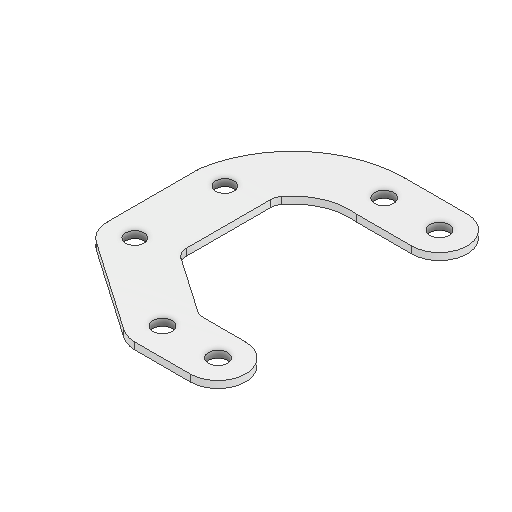
# Autodesk Inventor part: Rear Gusset
Saved by Autodesk Inventor 2025 (Build 290162000, 162)
## iProperties
Created: 2025-02-12
Part Number: Rear Gusset
Material: Acetal Resin, White
Document SubType Name: Modeling
Designer: Averey Ku
Density: 1.425 g/cm^3
Appearance: Smooth - White
Author: Averey Ku
Autodesk Inventor part; units mm, degrees
ref_plane "YZ Plane" through (0, 0, 0) normal (1, 0, 0) x (0, 1, 0)
ref_plane "XZ Plane" through (0, 0, 0) normal (0, 1, 0) x (-1, 0, 0)
ref_plane "XY Plane" through (0, 0, 0) normal (0, 0, 1) x (1, 0, 0)
sketch "gusset" plane through (0, 0, 0) normal (0, 0, 1) x (1, 0, 0)
  circle A0 centre (-8.9225, 14.8571) radius 2.1844
  circle A1 centre (-21.6225, 14.8571) radius 2.1844
  arc A2 (-21.6225, 21.2071) -> (-21.6225, 8.5071) centre (-21.6225, 14.8571) ccw
  arc A3 (-5.308, 20.078) -> (-8.9225, 21.2071) centre (-8.9225, 14.8571) ccw
  line L0 (18.065, 0.5696) -> (18.065, -20.0679)
  line L1 (3.7775, -22.5548) -> (3.7775, -3.322)
  line L2 (2.4097, -0.7116) -> (-10.0906, 7.9425)
  line L3 (-21.6225, 8.5071) -> (-11.8979, 8.5071)
  line L4 (-21.6225, 21.2071) -> (-8.9225, 21.2071)
  arc A4 (18.065, 0.5696) -> (15.3295, 5.7905) centre (11.715, 0.5696) ccw
  line L5 (-5.308, 20.078) -> (15.3295, 5.7905)
  circle A5 centre (-21.6232, -35.9429) radius 2.1844
  circle A6 centre (-8.9225, -35.9429) radius 2.1844
  line L6 (-21.6246, -29.5943) -> (-8.9205, -29.5916)
  line L7 (-21.6233, -42.2916) -> (-7.3358, -42.2916)
  arc A7 (-21.6246, -29.5943) -> (-21.6233, -42.2916) centre (-21.6232, -35.9429) ccw
  circle A8 centre (11.715, 0.5696) radius 2.0955
  circle A9 centre (11.715, -20.0679) radius 2.0955
  arc A10 (3.7775, -3.322) -> (2.4097, -0.7116) centre (0.6025, -3.322) ccw
  arc A11 (-10.0906, 7.9425) -> (-11.8979, 8.5071) centre (-11.8979, 5.3321) ccw
  arc A12 (-7.3358, -42.2916) -> (17.9607, -21.2138) centre (-7.3358, -16.5727) ccw
  arc A13 (17.9607, -21.2138) -> (18.065, -20.0679) centre (11.715, -20.0679) ccw
  arc A14 (-8.9205, -29.5916) -> (3.1382, -24.4655) centre (-7.3358, -16.5727) ccw
  arc A15 (3.1382, -24.4655) -> (3.7775, -22.5548) centre (0.6025, -22.5548) ccw
  point P0 (-7.0147, -10.522)
  point P1 (18.065, -20.6044)
  point P2 (3.7775, -23.5365)
  point P3 (5.0107, 12.9342)
  dimension "d0" = 12.7
  dimension "d2" = 14.2875
  dimension "d3" = 4.191
  dimension "d4" = 3.175
  dimension "d8" = 12.7
  dimension "d12" = 14.2875
  dimension "d13" = 6.35
  dimension "d14" = 15.875
  dimension "d15" = 3.175
  measures "d0" diameter of A4
  measures "d3" diameter of A8
  measures "d4" radius of A10
  measures "d8" distance from line of L2 point (5.011, 12.934)
  measures "d12" distance of L7.start L7.end
  measures "d13" radius of A13
  measures "d14" vertical distance of A6.centre A9.centre
  measures "d15" radius of A15
sketch "Sketch1" plane through (0, 0, 0) normal (0, 1, 0) x (-1, 0, 0)
  circle A0 centre (12.7, 0) radius 2.1844
  circle A1 centre (0, 0) radius 2.1844
  arc A2 (0, 6.35) -> (0, -6.35) centre (0, 0) ccw
  arc A3 (16.3145, 5.2209) -> (12.7, 6.35) centre (12.7, 0) ccw
  line L0 (39.6875, -14.2875) -> (39.6875, -34.925)
  line L1 (25.4, -37.4118) -> (25.4, -18.1791)
  line L2 (24.0322, -15.5687) -> (11.5319, -6.9145)
  line L3 (0, -6.35) -> (9.7246, -6.35)
  line L4 (0, 6.35) -> (12.7, 6.35)
  arc A4 (39.6875, -14.2875) -> (36.952, -9.0666) centre (33.3375, -14.2875) ccw
  line L5 (16.3145, 5.2209) -> (36.952, -9.0666)
  circle A5 centre (-0.0007, -50.8) radius 2.1844
  circle A6 centre (12.7, -50.8) radius 2.1844
  line L6 (-0.0021, -44.4514) -> (12.702, -44.4486)
  line L7 (-0.0008, -57.1486) -> (14.2867, -57.1486)
  arc A7 (-0.0021, -44.4514) -> (-0.0008, -57.1486) centre (-0.0007, -50.8) ccw
  circle A8 centre (33.3375, -14.2875) radius 2.0955
  circle A9 centre (33.3375, -34.925) radius 2.0955
  arc A10 (25.4, -18.1791) -> (24.0322, -15.5687) centre (22.225, -18.1791) ccw
  arc A11 (11.5319, -6.9145) -> (9.7246, -6.35) centre (9.7246, -9.525) ccw
  arc A12 (14.2867, -57.1486) -> (39.5833, -36.0709) centre (14.2867, -31.4298) ccw
  arc A13 (39.5833, -36.0709) -> (39.6875, -34.925) centre (33.3375, -34.925) ccw
  arc A14 (12.702, -44.4486) -> (24.7607, -39.3226) centre (14.2867, -31.4298) ccw
  arc A15 (24.7607, -39.3226) -> (25.4, -37.4118) centre (22.225, -37.4118) ccw
  constraints: 1 other
extrude "Extrusion1" add sketch "Sketch1" along normal blind 1.5875
body "Solid1"
